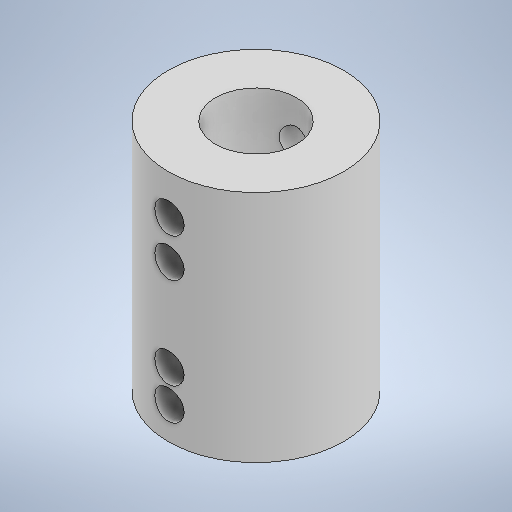
# Autodesk Inventor part: wellenkupplung_3mm_8mm
Saved by Autodesk Inventor 2025 (Build 290162000, 162)
## iProperties
Created: 2026-06-16
Part Number: wellenkupplung_3mm_8mm
Material: Generisch
Document SubType Name: Modeling
Designer: GemmiDad-GBSE
Density: 1 g/cm^3
Appearance: Vorgabe
Author: GemmiDad-GBSE
Autodesk Inventor part; units mm, degrees
ref_plane "YZ Plane" through (0, 0, 0) normal (1, 0, 0) x (0, 1, 0)
ref_plane "XZ Plane" through (0, 0, 0) normal (0, 1, 0) x (-1, 0, 0)
sketch "Skizze1" plane through (0, 0, 0) normal (0, 0, 1) x (1, 0, 0)
  circle A0 centre (0, 0) radius 9
  constraints: 1 centre point
extrude "Extrusion1" add sketch "Skizze1" along normal blind 24
sketch "Skizze2" plane through (0, 0, 0) normal (0, 0, 1) x (1, 0, 0)
  circle A0 centre (0, 0) radius 1.6
  constraints: 1 centre point
extrude "Extrusion2" cut sketch "Skizze2" along normal blind 10
ref_plane "Arbeitsebene1" through (0, 0, 24) normal (0, 0, 1) x (1, 0, 0)
sketch "Skizze3" plane through (0, 0, 24) normal (0, 0, 1) x (1, 0, 0)
  circle A0 centre (0, 0) radius 4.15
  constraints: 1 centre point
extrude "Extrusion3" cut sketch "Skizze3" against normal blind 12
sketch "Skizze4" plane through (0, 0, 0) normal (0, 1, 0) x (-1, 0, 0)
  circle A0 centre (0, 3.3) radius 1.5
  circle A1 centre (0, 6.6) radius 1.5
  circle A2 centre (0, 15.96) radius 1.5
  circle A3 centre (0, 19.92) radius 1.5
  constraints: 4 centre point
extrude "Extrusion4" cut sketch "Skizze4" along normal mid plane 18
